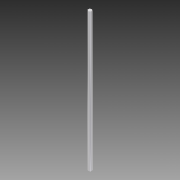
# Autodesk Inventor part: varilla 10 carro y
Saved by Autodesk Inventor 2012 (Build 160160000, 160)
## iProperties
Created: 2014-07-04
Part Number: varilla 10 carro y
Material: Default
Document SubType Name: Modeling
Designer: Principal
Density: 1 g/cm^3
Author: Principal
Autodesk Inventor part; units mm, degrees
ref_plane "YZ Plane" through (0, 0, 0) normal (1, 0, 0) x (0, 1, 0)
ref_plane "XZ Plane" through (0, 0, 0) normal (0, 1, 0) x (-1, 0, 0)
ref_plane "XY Plane" through (0, 0, 0) normal (0, 0, 1) x (1, 0, 0)
sketch "Boceto1" plane through (0, 0, 0) normal (0, 0, 1) x (1, 0, 0)
  circle A0 centre (0, 0) radius 5
  constraints: 1 centre point, 1 coincident
extrude "Extrusión1" add sketch "Boceto1" along normal blind 397.8
fillet "Empalme1" radius 0.5 2 edges at (-5, 0, 397.8) (-5, 0, 0)
